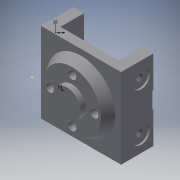
# Autodesk Inventor part: polaczenie_CH-R
Saved by Autodesk Inventor 2017 (Build 210142000, 142)
## iProperties
Created: 2017-10-30
Part Number: polaczenie_CH-R
Material: Ogólny
Document SubType Name: Modeling
Designer: Michał Spławski
Density: 1 g/cm^3
Appearance: Domyślna
Author: Michał Spławski
Autodesk Inventor part; units mm, degrees
ref_plane "YZ Plane" through (0, 0, 0) normal (1, 0, 0) x (0, 1, 0)
ref_plane "XZ Plane" through (0, 0, 0) normal (0, 1, 0) x (-1, 0, 0)
ref_plane "XY Plane" through (0, 0, 0) normal (0, 0, 1) x (1, 0, 0)
sketch "Szkic1" plane through (0, 0, 0) normal (0, 1, 0) x (-1, 0, 0)
  circle A0 centre (0, 0) radius 32.5
  dimension "d0" = 65
  constraints: 1 centre point, 1 coincident
  measures "d0" diameter of A0
extrude "Wyciągnięcie proste1" add sketch "Szkic1" along normal blind 10
sketch "Szkic2" plane through (0, 10, 0) normal (0, 1, 0) x (1, 0, 0)
  circle A0 centre (0, 0) radius 15.75
  circle A1 centre (0, 25) radius 4.75
  circle A2 centre (-25, 0) radius 4.75
  circle A3 centre (0, -25) radius 4.75
  circle A4 centre (25, 0) radius 4.75
  dimension "d3" = 31.5
  dimension "d4" = 9.5
  dimension "d5" = 25
  dimension "d8" = 360
  constraints: 5 centre point, 3 coincident, 1 vertical alignment, 11 other
  measures "d3" diameter of A0
  measures "d4" diameter of A1
  measures "d5" distance of point (0, 0) A1.centre
extrude "Wyciągnięcie proste2" cut sketch "Szkic2" against normal blind 23.25 contours A1 | A2 | A3 | A4
sketch "Szkic3" plane through (0, 0, 0) normal (0, -1, 0) x (1, 0, 0)
  circle A0 centre (0, 0) radius 15.75
  dimension "d12" = 31.5
  constraints: 1 centre point, 1 coincident
  measures "d12" diameter of A0
extrude "Wyciągnięcie proste3" add sketch "Szkic3" along normal blind 6
sketch "Szkic4" plane through (0, 10, 0) normal (0, 1, 0) x (1, 0, 0)
  line L0 (-45, 45) -> (45, 45)
  line L1 (45, 45) -> (45, -45)
  line L2 (45, -45) -> (-45, -45)
  line L3 (-45, -45) -> (-45, 45)
  point P0 (0, 0)
  point P1 (0, 45)
  point P2 (45, 0)
  dimension "d15" = 90
  dimension "d16" = 90
  constraints: 8 end point, 2 midpoint, 2 parallel, 1 horizontal, 1 horizontal alignment, 1 perpendicular, 1 vertical alignment
  measures "d15" distance of L0.start L0.end
  measures "d16" distance of L0.end L1.end
extrude "Wyciągnięcie proste4" add sketch "Szkic4" along normal blind 10
sketch "Szkic5" plane through (0, 10, 0) normal (0, -1, 0) x (1, 0, 0)
  circle A0 centre (-25, 0) radius 4.75 projected
  circle A1 centre (0, 25) radius 4.75 projected
  circle A2 centre (25, 0) radius 4.75 projected
  circle A3 centre (0, -25) radius 4.75 projected
  point P0 (0, 0)
extrude "Wyciągnięcie proste5" cut sketch "Szkic5" along normal mid plane 50
sketch "Szkic6" plane through (0, 20, 0) normal (0, 1, 0) x (1, 0, 0)
  circle A0 centre (0, 25) radius 4.75 projected
  circle A1 centre (25, 0) radius 4.75 projected
  circle A2 centre (-25, 0) radius 4.75 projected
  circle A3 centre (0, -25) radius 4.75 projected
  circle A4 centre (-25, 0) radius 9.25
  circle A5 centre (0, 0) radius 15.75 projected
  circle A6 centre (0, 25) radius 9.25
  circle A7 centre (25, 0) radius 4.75 projected
  circle A8 centre (25, 0) radius 9.25
  circle A9 centre (0, -25) radius 9.25
  constraints: 4 centre point, 4 coincident, 4 tangent
extrude "Wyciągnięcie proste6" cut sketch "Szkic6" against normal blind 4 contours A4 | A6 | A8 | A9
sketch "Szkic7" plane through (0, 10, 0) normal (0, -1, 0) x (1, 0, 0)
  circle A0 centre (0, 0) radius 38.5
  dimension "d29" = 77
  constraints: 1 centre point, 1 coincident
  measures "d29" diameter of A0
sketch "Szkic8" plane through (0, 0, 0) normal (0, -1, 0) x (1, 0, 0)
  circle A0 centre (0, 0) radius 32.5
  constraints: 1 centre point, 1 coincident
loft "Wyciągnięcie złożone1" add profiles "Szkic7" section 2 edges at (32.5, 0, 0)
sketch "Szkic9" plane through (0, 0, 0) normal (0, -1, 0) x (1, 0, 0)
  circle A0 centre (0, -25) radius 4.75 projected
  circle A1 centre (-25, 0) radius 4.75 projected
  circle A2 centre (0, 25) radius 4.75 projected
  circle A3 centre (25, 0) radius 4.75 projected
  point P0 (0, 0)
extrude "Wyciągnięcie proste7" cut sketch "Szkic9" against normal blind 30
sketch "Szkic10" plane through (0, 20, 0) normal (0, 1, 0) x (1, 0, 0)
  line L0 (-45, -45) -> (-45, 45) projected
  line L1 (-45, -45) -> (-33, -45)
  line L2 (-33, -45) -> (-33, -9)
  line L3 (-33, -9) -> (-45, -9)
  line L4 (-45, -9) -> (-45, -45)
  line L5 (-45, 45) -> (-32.5, 45)
  line L6 (-32.5, 45) -> (-32.5, 9)
  line L7 (-32.5, 9) -> (-45, 9)
  line L8 (-45, 9) -> (-45, 45)
  line L9 (45, -45) -> (-45, -45) projected
  line L10 (45, -45) -> (33, -45)
  line L11 (33, -45) -> (33, -9)
  line L12 (33, -9) -> (45, -9)
  line L13 (45, -9) -> (45, -45)
  line L14 (45, 45) -> (33, 45)
  line L15 (33, 45) -> (33, 9)
  line L16 (33, 9) -> (45, 9)
  line L17 (45, 9) -> (45, 45)
  point P0 (0, 0)
  dimension "d30" = 12
  dimension "d31" = 36
  constraints: 32 end point, 8 parallel, 4 horizontal, 4 perpendicular, 4 point on line
  measures "d30" distance of L3.end L2.end
  measures "d31" distance of L5.end L6.end
extrude "Wyciągnięcie proste8" add sketch "Szkic10" along normal blind 26.325
sketch "Szkic11" plane through (45, 10, 45) normal (1, 0, 0) x (0, 0, -1)
  circle A0 centre (18, 22.5) radius 5
  circle A1 centre (72, 22.5) radius 5
  point P0 (45, -10)
  dimension "d34" = 10
  dimension "d35" = 10
  constraints: 2 centre point
  measures "d34" diameter of A0
  measures "d35" diameter of A1
sketch "Szkic12" plane through (-45, 10, -45) normal (-1, 0, 0) x (0, 0, 1)
  circle A0 centre (18, 22.5) radius 5
  circle A1 centre (72, 22.5) radius 5
  point P0 (45, -10)
  dimension "d36" = 10
  dimension "d37" = 10
  constraints: 2 centre point
  measures "d36" diameter of A0
  measures "d37" diameter of A1
sketch "Szkic13" plane through (-45, 10, -45) normal (-1, 0, 0) x (0, 0, 1)
  point P0 (45, -10)
sketch "Szkic14" plane through (-45, 10, -45) normal (-1, 0, 0) x (0, 0, 1)
  line L0 (36, 10) -> (54, 10) projected
  line L1 (36, 10) -> (54, 10)
  line L2 (54, 10) -> (54, 36)
  line L3 (54, 36) -> (36, 36)
  line L4 (36, 36) -> (36, 10)
  point P0 (45, -10)
  constraints: 8 end point, 2 parallel, 1 horizontal, 1 perpendicular
extrude "Wyciągnięcie proste9" add sketch "Szkic14" against normal blind 10
sketch "Szkic15" plane through (45, 10, 45) normal (1, 0, 0) x (0, 0, -1)
  line L0 (36, 10) -> (36, 36.325) projected
  line L1 (54, 10) -> (54, 36.325) projected
  line L2 (36, 10) -> (54, 10)
  line L3 (54, 10) -> (54, 35)
  line L4 (54, 35) -> (36, 35)
  line L5 (36, 35) -> (36, 10)
  point P0 (45, -10)
  constraints: 8 end point, 2 parallel, 1 horizontal, 1 perpendicular, 1 point on line
extrude "Wyciągnięcie proste10" add sketch "Szkic15" against normal blind 10
hole "Otwór1" at (45, 32.5, 27) at (45, 32.5, -27) direction (-1, 0, 0) diameter 7.188 depth 24 tip angle 118 counterbore diameter 18 counterbore depth 4 thread size "M8x0.75" class "6H" standard "ISO Metric profile"
hole "Otwór2" at (-45, 32.5, -27) at (-45, 32.5, 27) direction (1, 0, 0) diameter 7.188 depth 20 tip angle 118 counterbore diameter 18 counterbore depth 4 thread size "M8x0.75" class "6H" standard "ISO Metric profile"
